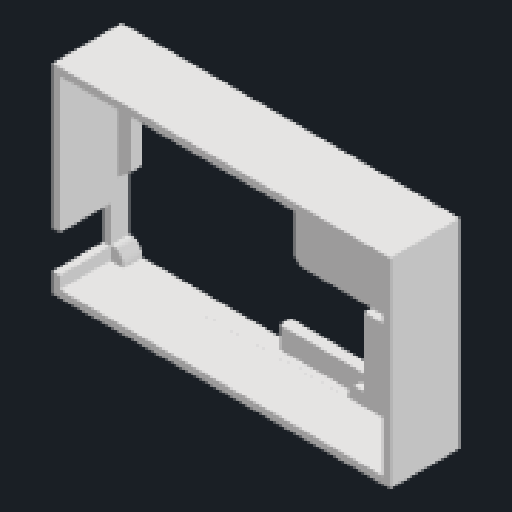
# Autodesk Inventor part: Buttom_case
Saved by Autodesk Inventor 2026.2 (Build 302298000, 298)
## iProperties
Created: 2026-04-11
Part Number: Buttom_case
Material: Generic
Document SubType Name: Modeling
Designer: Malthe Sennels
Density: 1 g/cm^3
Appearance: Default
Author: Malthe Sennels
Autodesk Inventor part; units mm, degrees
ref_plane "YZ Plane" through (0, 0, 0) normal (1, 0, 0) x (0, 1, 0)
ref_plane "XZ Plane" through (0, 0, 0) normal (0, 1, 0) x (-1, 0, 0)
sketch "Sketch1" plane through (0, 0, 0) normal (0, 0, 1) x (1, 0, 0)
  line L0 (139.954, -59.944) -> (184.404, -59.944)
  arc A0 (136.4, -63.498) -> (139.954, -59.944) centre (136.4, -59.944) ccw
  line L1 (136.398, -104.648) -> (136.4, -63.498)
  arc A1 (139.952, -108.202) -> (136.398, -104.648) centre (136.398, -108.202) ccw
  line L2 (198.6031, -108.1771) -> (139.952, -108.202)
  arc A2 (202.184, -104.6232) -> (198.6031, -108.1771) centre (202.1571, -108.1771) ccw
  line L3 (187.185, -59.444) -> (139.4128, -59.444)
  arc A3 (135.9, -62.9568) -> (139.4128, -59.444) centre (136.4, -59.944) ccw
  line L4 (135.9, -62.9568) -> (135.898, -105.1892)
  arc A4 (139.4108, -108.7022) -> (135.898, -105.1892) centre (136.398, -108.202) ccw
  line L5 (139.4108, -108.7022) -> (199.1442, -108.6768)
  arc A5 (202.1802, -105.1231) -> (199.1442, -108.6768) centre (202.1571, -108.1771) ccw
  line L6 (187.185, -59.444) -> (224.685, -59.444)
  line L7 (224.685, -59.444) -> (224.685, -105.1231)
  line L8 (224.685, -105.1231) -> (202.1802, -105.1231)
  line L9 (133.9, -57.444) -> (226.685, -57.444)
  line L10 (226.685, -57.444) -> (226.685, -110.6768)
  line L11 (226.685, -110.6768) -> (133.9, -110.6768)
  line L12 (133.9, -110.6768) -> (133.9, -57.444)
  line L13 (224.685, -105.1231) -> (206.185, -105.1231)
  line L14 (206.185, -105.1231) -> (206.185, -86.9231)
  line L15 (206.185, -86.9231) -> (224.685, -86.9231)
  line L16 (224.685, -86.9231) -> (224.685, -105.1231)
  line L17 (225.185, -101.396) -> (225.185, -85.896)
  line L18 (224.685, -59.444) -> (221.285, -59.444)
  line L19 (221.285, -59.444) -> (221.285, -67.444)
  line L20 (221.285, -67.444) -> (224.685, -67.444)
  line L21 (224.685, -67.444) -> (224.685, -59.444)
  point P0 (0, 0)
extrude "Extrusion1" add sketch "Sketch1" against normal blind 2 contours L6 L7 L20 L19 | L7 L8 L14 L15 | L9 L10 L11 L12
sketch "Sketch2" plane through (0, 0, -2) normal (0, 0, -1) x (-1, 0, 0)
  line L0 (-226.685, -110.6768) -> (-133.9, -110.6768) projected
  line L1 (-133.9, -110.6768) -> (-133.9, -57.444) projected
  line L2 (-133.9, -57.444) -> (-226.685, -57.444) projected
  line L3 (-226.685, -57.444) -> (-226.685, -110.6768) projected
  line L4 (-221.285, -59.444) -> (-139.4128, -59.444) projected
  arc A0 (-139.4128, -59.444) -> (-135.9, -62.9568) centre (-136.4, -59.944) ccw projected
  line L5 (-135.9, -62.9568) -> (-135.898, -105.1892) projected
  arc A1 (-135.898, -105.1892) -> (-139.4108, -108.7022) centre (-136.398, -108.202) ccw projected
  line L6 (-139.4108, -108.7022) -> (-199.1442, -108.6768) projected
  arc A2 (-199.1442, -108.6768) -> (-202.1802, -105.1231) centre (-202.1571, -108.1771) ccw projected
  line L7 (-202.1802, -105.1231) -> (-206.185, -105.1231) projected
  line L8 (-206.185, -105.1231) -> (-206.185, -86.9231) projected
  line L9 (-206.185, -86.9231) -> (-224.685, -86.9231) projected
  line L10 (-224.685, -86.9231) -> (-224.685, -67.444) projected
  line L11 (-206.185, -101.9751) -> (-181.6826, -101.9751)
  line L12 (-181.6826, -101.9751) -> (-181.6854, -108.6843)
  line L13 (-177.0715, -59.444) -> (-182.7923, -64.1474)
  line L14 (-182.7923, -64.1474) -> (-182.7923, -84.0815)
  line L15 (-182.7923, -84.0815) -> (-185.4081, -86.9231)
  line L16 (-185.4081, -86.9231) -> (-206.185, -86.9231)
  line L17 (-135.8997, -70.5788) -> (-139.4108, -73.1836)
  line L18 (-139.4108, -73.1836) -> (-139.4108, -87.5874)
  line L19 (-139.4108, -87.5874) -> (-135.8987, -90.4582)
  line L20 (-182.7923, -79.0709) -> (-188.2357, -79.0709)
  arc A3 (-190.4025, -77.0764) -> (-188.2357, -79.0709) centre (-188.2357, -76.8967) ccw
  line L21 (-190.4025, -77.0764) -> (-190.4025, -68.8146)
  arc A4 (-187.5463, -65.9584) -> (-190.4025, -68.8146) centre (-187.5463, -68.8146) ccw
  line L22 (-187.5463, -65.9584) -> (-182.7923, -65.9584)
  line L23 (-226.685, -57.444) -> (-221.285, -57.444)
  line L24 (-221.285, -57.444) -> (-221.285, -65.444)
  line L25 (-221.285, -65.444) -> (-226.685, -65.444)
  line L26 (-226.685, -65.444) -> (-226.685, -57.444)
  line L27 (-224.685, -67.444) -> (-221.285, -67.444) projected
  line L28 (-221.285, -67.444) -> (-221.285, -59.444) projected
  point P0 (0, 0)
  dimension "d47" = 5.4
  dimension "d48" = 8
  constraints: 32 end point, 7 point on line, 4 horizontal, 4 perpendicular, 4 point on circle, 3 tangent, 2 centre point, 2 parallel, 2 vertical
  measures "d47" distance of L24.end L25.end
  measures "d48" distance of L23.end L24.end
extrude "Extrusion2" add sketch "Sketch2" along normal blind 3 contours L3 L25 L28 L27 L10 L9 L8 L7 A2 L6 A1 L5 A0 L4 L24 L2 L1 L0 | L3 L2 L24 L25 | L24 L4 L13 L14 L22 A4 L21 A3 L20 L15 L16 L9 L10 L27 L28 | L5 L19 L18 L17 | L11 L12 L6 A2 L7 L8
sketch "Sketch3" plane through (0, 0, 0) normal (0, 0, 1) x (1, 0, 0)
  line L0 (133.9, -110.6768) -> (226.685, -110.6768) projected
  line L1 (226.685, -110.6768) -> (226.685, -57.444) projected
  line L2 (226.685, -57.444) -> (133.9, -57.444) projected
  line L3 (133.9, -57.444) -> (133.9, -110.6768) projected
  line L4 (139.4128, -59.444) -> (221.285, -59.444) projected
  line L5 (224.685, -67.444) -> (224.685, -86.9231) projected
  line L6 (224.685, -86.9231) -> (206.185, -86.9231) projected
  line L7 (206.185, -86.9231) -> (206.185, -105.1231) projected
  line L8 (206.185, -105.1231) -> (202.1802, -105.1231) projected
  arc A0 (202.1802, -105.1231) -> (199.1442, -108.6768) centre (202.1571, -108.1771) ccw projected
  line L9 (199.1442, -108.6768) -> (139.4108, -108.7022) projected
  arc A1 (139.4108, -108.7022) -> (135.898, -105.1892) centre (136.398, -108.202) ccw projected
  line L10 (135.898, -105.1892) -> (135.9, -62.9568) projected
  arc A2 (135.9, -62.9568) -> (139.4128, -59.444) centre (136.4, -59.944) ccw projected
  line L11 (133.9, -57.444) -> (226.685, -57.444)
  line L12 (226.685, -57.444) -> (226.685, -110.6768)
  line L13 (226.685, -110.6768) -> (133.9, -110.6768)
  line L14 (133.9, -110.6768) -> (133.9, -57.444)
  line L15 (135.9, -59.444) -> (224.685, -59.444)
  line L16 (224.685, -59.444) -> (224.685, -108.7022)
  line L17 (224.685, -108.7022) -> (135.9, -108.7022)
  line L18 (135.9, -108.7022) -> (135.9, -59.444)
  line L19 (135.989, -96.1155) -> (132.989, -96.1155) projected
  line L20 (135.989, -104.9155) -> (132.989, -104.9155) projected
  line L21 (135.989, -95.6155) -> (132.989, -95.6155)
  line L22 (135.989, -105.4155) -> (132.989, -105.4155)
  line L23 (133.3303, -95.6155) -> (137.6479, -95.6155)
  line L24 (137.6479, -95.6155) -> (137.6479, -105.4155)
  line L25 (137.6479, -105.4155) -> (133.3303, -105.4155)
  line L26 (133.3303, -105.4155) -> (133.3303, -95.6155)
  line L27 (226.685, -57.444) -> (221.285, -57.444)
  line L28 (221.285, -57.444) -> (221.285, -65.444)
  line L29 (221.285, -65.444) -> (226.685, -65.444)
  line L30 (226.685, -65.444) -> (226.685, -57.444)
  line L31 (221.285, -59.444) -> (221.285, -67.444) projected
  line L32 (221.285, -67.444) -> (224.685, -67.444) projected
  point P0 (0, 0)
  point P1 (135.9, -105.4155)
  point P2 (133.9, -105.4155)
  point P3 (133.9, -95.6155)
  point P4 (135.8984, -95.6155)
  point P5 (224.685, -59.444)
  point P6 (221.904, -86.9231)
  point P7 (135.9, -105.1889)
  point P8 (135.9, -95.6155)
  point P9 (221.285, -59.444)
  point P10 (135.898, -104.9155)
  point P11 (135.9, -104.9155)
  dimension "d12" = 0.5
  dimension "d13" = 0.5
  dimension "d45" = 5.4
  dimension "d46" = 8
  constraints: 36 end point, 10 parallel, 4 horizontal, 4 perpendicular, 2 point on line, 1 point on circle
  measures "d12" distance between parallel lines of L19 L21
  measures "d13" distance between parallel lines of L20 L22
  measures "d45" distance of L29.end L28.end
  measures "d46" distance of L28.end L27.end
extrude "Extrusion3" add sketch "Sketch3" along normal blind 15 from surface at 0 contours L3 L22 L18 L17 L16 L5 L29 L1 L0 | L29 L16 L15 L28 L2 L1 | L22 L25 A1 L17 L18 | L29 L28 L15 L16 | L16 L32 L31 L29 | L28 L4 L15 L18 L10 L21 L3 L2 | A2 L18 L15
sketch "Sketch4" plane through (0, 0, -5) normal (0, 0, -1) x (-1, 0, 0)
  line L0 (-133.9, -110.6768) -> (-133.9, -57.444) projected
  line L1 (-133.9, -57.444) -> (-226.685, -57.444) projected
  line L2 (-226.685, -57.444) -> (-226.685, -110.6768) projected
  line L3 (-226.685, -110.6768) -> (-133.9, -110.6768) projected
  arc A0 (-139.4128, -59.444) -> (-135.9, -62.9568) centre (-136.4, -59.944) ccw projected
  line L4 (-135.9, -62.9568) -> (-135.8997, -70.5788) projected
  line L5 (-135.8997, -70.5788) -> (-139.4108, -73.1836) projected
  line L6 (-139.4108, -73.1836) -> (-139.4108, -87.5874) projected
  line L7 (-139.4108, -87.5874) -> (-135.8987, -90.4582) projected
  line L8 (-135.8987, -90.4582) -> (-135.898, -105.1892) projected
  arc A1 (-135.898, -105.1892) -> (-139.4108, -108.7022) centre (-136.398, -108.202) ccw projected
  line L9 (-139.4108, -108.7022) -> (-181.6854, -108.6843) projected
  line L10 (-181.6854, -108.6843) -> (-181.6826, -101.9751) projected
  line L11 (-181.6826, -101.9751) -> (-206.185, -101.9751) projected
  line L12 (-206.185, -101.9751) -> (-206.185, -86.9231) projected
  line L13 (-206.185, -86.9231) -> (-185.4081, -86.9231) projected
  line L14 (-185.4081, -86.9231) -> (-182.7923, -84.0815) projected
  line L15 (-182.7923, -84.0815) -> (-182.7923, -79.0709) projected
  line L16 (-182.7923, -79.0709) -> (-188.2357, -79.0709) projected
  arc A2 (-190.4025, -77.0764) -> (-188.2357, -79.0709) centre (-188.2357, -76.8967) ccw projected
  line L17 (-190.4025, -77.0764) -> (-190.4025, -68.8146) projected
  arc A3 (-187.5463, -65.9584) -> (-190.4025, -68.8146) centre (-187.5463, -68.8146) ccw projected
  line L18 (-187.5463, -65.9584) -> (-182.7923, -65.9584) projected
  line L19 (-182.7923, -65.9584) -> (-182.7923, -64.1474) projected
  line L20 (-182.7923, -64.1474) -> (-177.0715, -59.444) projected
  line L21 (-177.0715, -59.444) -> (-139.4128, -59.444) projected
  point P0 (0, 0)
extrude "Extrusion4" add sketch "Sketch4" along normal blind 2 contours L3 L2 L1 L0 | A0 L4 L5 L6 L7 L8 A1 L9 L10 L11 L12 L13 L14 L15 L16 A2 L17 A3 L18 L19 L20 L21
sketch "Sketch5" plane through (133.9, -105.4155, 0) normal (-1, 0, 0) x (0, 0, 1)
  line L0 (8.585, 34.6765) -> (8.585, 37.2165) projected
  line L1 (8.585, 11.8165) -> (8.585, 14.3565) projected
  line L2 (6.585, 30.3855) -> (22, 30.3855)
  line L3 (22, 30.3855) -> (22, 18.3855)
  line L4 (22, 18.3855) -> (6.585, 18.3855)
  line L5 (6.585, 18.3855) -> (6.585, 30.3855)
  line L6 (6.585, 24.3855) -> (22, 24.3855)
  line L7 (6.585, 30.3855) -> (15, 30.3855)
  line L8 (15, 30.3855) -> (15, 18.3855)
  line L9 (15, 18.3855) -> (6.585, 18.3855)
  line L10 (15, 42.4587) -> (15, 9.8) projected
  line L11 (22, 18.3855) -> (22, 30.3855)
  line L12 (-8.585, -34.6765) -> (-8.585, -37.2165) projected
  line L13 (-8.585, -11.8165) -> (-8.585, -14.3565) projected
  line L14 (22, 18.3855) -> (24, 18.3855)
  line L15 (24, 18.3855) -> (24, 30.3855)
  line L16 (24, 30.3855) -> (22, 30.3855)
  line L17 (22, 30.3855) -> (22, 18.3855)
  point P0 (0, 105.4155)
  point P1 (14.2925, 18.3855)
  point P2 (16.8, 24.3855)
  point P3 (15, -30.5165)
  point P4 (15, 47.9715)
  point P5 (22, 30.3855)
  point P6 (15, 18.3855)
  dimension "d19" = 20.32
  dimension "d22" = 7
  dimension "d23" = 1.8
  dimension "d51" = 2
  dimension "d52" = 2
  constraints: 26 end point, 4 parallel, 4 perpendicular, 3 horizontal, 3 midpoint, 2 point on line
  measures "d19" distance of L0.start L1.end
  measures "d22" distance between parallel lines of L8 L3
  measures "d23" distance from line of point (16.8, 24.386) L8
  measures "d51" distance of L16.end L15.end
  measures "d52" distance between parallel lines of L0 L5
extrude "Extrusion5" cut sketch "Sketch5" against normal blind 16
fillet "Fillet1" radius 2 2 edges at (134.8994, -87.03, 6.585) (134.8997, -75.03, 6.585)
sketch "Sketch6" plane through (224.685, -86.9231, -2) normal (-1, 0, 0) x (0, 0, 1)
  circle A0 centre (20.335, -6.7229) radius 2.65 projected
  circle A1 centre (20.335, -6.7229) radius 3.35
  line L0 (17, -21.7791) -> (17, 19.4791) projected
  line L1 (17, 5.2771) -> (25, -2.7229)
  line L2 (25, -2.7229) -> (25, -10.7229)
  line L3 (25, -10.7229) -> (17, -18.7229)
  point P0 (2, 86.9231)
  point P1 (17, 27.4791)
  point P2 (17, -6.4062)
  point P3 (17, -7.0395)
  dimension "d27" = 0.7
  dimension "d28" = 45
  dimension "d29" = 45
  dimension "d30" = 8
  dimension "d31" = 4
  dimension "d32" = 4
  constraints: 6 end point, 2 point on line, 1 centre point, 1 parallel
  measures "d27" radial gap between concentric circles of A0 A1
  measures "d28" angle of L3 L0
  measures "d29" angle of L1 L0
  measures "d30" distance between parallel lines of L2 L0
  measures "d31" vertical distance of L2.end A0.centre
  measures "d32" vertical distance of L1.end A0.centre
extrude "Extrusion6" add sketch "Sketch6" against normal up to surface (2 mm away) contours A1 L0 L1 L2 L3
sketch "Sketch8" plane through (0, 0, 0) normal (0, 0, 1) x (1, 0, 0)
  line L0 (224.685, -108.7022) -> (224.685, -86.9231) projected
  line L1 (224.685, -108.7022) -> (220.685, -108.7022)
  line L2 (220.685, -108.7022) -> (220.685, -103.7022)
  line L3 (220.685, -103.7022) -> (224.685, -103.7022)
  line L4 (224.685, -103.7022) -> (224.685, -108.7022)
  point P0 (0, 0)
  dimension "d57" = 4
  dimension "d58" = 5
  constraints: 8 end point, 2 parallel, 1 horizontal, 1 perpendicular
  measures "d57" distance of L2.end L3.end
  measures "d58" distance of L1.end L2.end
extrude "Extrusion8" add sketch "Sketch8" along normal up to surface (15 mm away)
sketch "Sketch7" plane through (133.9, -57.444, 15) normal (0, 0, 1) x (1, 0, 0)
  circle A0 centre (1.3, -1.3) radius 1.8
  circle A1 centre (1.3, -1.3) radius 3.8
  line L0 (0, 0) -> (92.785, 0) projected
  line L1 (0, -53.2328) -> (0, 0) projected
  circle A2 centre (1.3, -51.9328) radius 1.8
  circle A3 centre (1.3, -51.9328) radius 3.8
  line L2 (92.785, -53.2328) -> (0, -53.2328) projected
  line L3 (0, -53.2328) -> (0, 0) projected
  line L4 (0, -47.9715) -> (3.7479, -47.9715) projected
  line L5 (92.785, -48.202) -> (90.785, -48.202) projected
  line L6 (0, -53.2328) -> (0, -47.9715) projected
  line L7 (92.785, -53.2328) -> (0, -53.2328) projected
  line L8 (92.785, -48.202) -> (92.785, -53.2328) projected
  line L9 (92.785, -35.8853) -> (90.785, -35.8853) projected
  line L10 (90.785, -24.202) -> (90.785, -10) projected
  line L11 (90.785, -24.202) -> (92.785, -24.202) projected
  line L12 (92.785, 0) -> (92.785, -24.202) projected
  line L13 (0, 0) -> (92.785, 0) projected
  line L14 (90.785, -36.5187) -> (92.785, -36.5187) projected
  line L15 (92.785, -35.8853) -> (92.785, -36.5187) projected
  line L16 (90.785, -36.5187) -> (90.785, -35.8853) projected
  line L17 (5.5107, -51.2582) -> (86.785, -51.2582) projected
  line L18 (1.9984, -38.1715) -> (0, -38.1715) projected
  line L19 (87.385, -2) -> (5.5128, -2) projected
  line L20 (87.385, -10) -> (87.385, -2) projected
  line L21 (90.785, -10) -> (87.385, -10) projected
  line L22 (0, -17.586) -> (0, 0) projected
  line L23 (2, -5.5128) -> (1.9994, -17.586) projected
  line L24 (0, -47.9715) -> (3.7479, -47.9715) projected
  line L25 (1.9988, -29.586) -> (0, -29.586) projected
  line L26 (0, -38.1715) -> (0, -29.586) projected
  line L27 (1.9988, -29.586) -> (1.9984, -38.1715) projected
  line L28 (0, -17.586) -> (1.9994, -17.586) projected
  arc A4 (2, -5.5128) -> (5.5128, -2) centre (2.5, -2.5) ccw projected
  arc A5 (5.5107, -51.2582) -> (3.7479, -47.9715) centre (2.498, -50.758) ccw projected
  circle A6 centre (91.485, -1.3) radius 1.8
  circle A7 centre (91.485, -1.3) radius 3.8
  line L29 (90.785, -46.2582) -> (90.785, -48.202) projected
  line L30 (86.785, -46.2582) -> (90.785, -46.2582) projected
  line L31 (86.785, -51.2582) -> (86.785, -46.2582) projected
  circle A8 centre (91.485, -51.9328) radius 1.8
  circle A9 centre (91.485, -51.9328) radius 3.8
  point P0 (-133.9, 57.444)
  point P1 (0, -17.455)
  point P2 (-20.1767, -7.6209)
  point P3 (0, -50.6878)
  point P4 (0, -53.1778)
  point P5 (0.055, -53.2328)
  point P6 (2.545, -53.2328)
  point P7 (0, -0.055)
  point P8 (0, -2.545)
  point P9 (2.545, 0)
  point P10 (0.055, 0)
  point P11 (2, -47.9715)
  point P12 (90.24, 0)
  point P13 (92.785, -2.545)
  point P14 (92.785, -50.7174)
  point P15 (92.785, -50.6878)
  point P16 (90.24, -53.2328)
  dimension "d35" = 3.6
  dimension "d36" = 2
  dimension "d37" = 1.3
  dimension "d38" = 1.3
  dimension "d39" = 3.6
  dimension "d40" = 2
  dimension "d41" = 1.3
  dimension "d42" = 1.3
  dimension "d53" = 3.6
  dimension "d54" = 2
  dimension "d55" = 1.3
  dimension "d56" = 1.3
  dimension "d61" = 3.6
  dimension "d62" = 2
  dimension "d63" = 1.3
  dimension "d64" = 1.3
  constraints: 8 centre point, 4 coincident, 1 midpoint
  measures "d35" diameter of A0
  measures "d36" radial gap between concentric circles of A1 A0
  measures "d37" distance from line of L0 A0.centre
  measures "d38" distance from line of L1 A0.centre
  measures "d39" diameter of A2
  measures "d40" radial gap between concentric circles of A3 A2
  measures "d41" distance from line of L2 A2.centre
  measures "d42" distance from line of L3 A2.centre
  measures "d53" diameter of A6
  measures "d54" radial gap between concentric circles of A6 A7
  measures "d55" distance from line of L12 A6.centre
  measures "d56" distance from line of L0 A6.centre
  measures "d61" diameter of A8
  measures "d62" radial gap between concentric circles of A8 A9
  measures "d63" horizontal distance of point (92.785, -50.717) A8.centre
  measures "d64" distance from line of L7 A8.centre
extrude "Extrusion7" cut sketch "Sketch7" against normal blind 25.6 contours A0 L1 L0 | A0 L1 L0 | L0 A6 L12 | L0 L12 A6 | L1 A2 L2 | L1 A2 L2 | A8 L8 L2 | A8 L8 L2
sketch "Sketch9" plane through (0, 0, -7) normal (0, 0, -1) x (-1, 0, 0)
  arc A0 (-136.445, -57.444) -> (-133.9, -59.989) centre (-135.2, -58.744) ccw projected
  arc A1 (-133.9, -108.1318) -> (-136.445, -110.6768) centre (-135.2, -109.3768) ccw projected
  arc A2 (-224.14, -110.6768) -> (-226.685, -108.1318) centre (-225.385, -109.3768) ccw projected
  arc A3 (-226.685, -59.989) -> (-224.14, -57.444) centre (-225.385, -58.744) ccw projected
  circle A4 centre (-225.385, -58.744) radius 3.8
  circle A5 centre (-225.385, -58.744) radius 1.8
  circle A6 centre (-225.385, -109.3768) radius 1.8
  circle A7 centre (-225.385, -109.3768) radius 3.8
  circle A8 centre (-135.2, -58.744) radius 1.8
  circle A9 centre (-135.2, -58.744) radius 3.8
  circle A10 centre (-135.2, -109.3768) radius 1.8
  circle A11 centre (-135.2, -109.3768) radius 3.8
  point P0 (0, 0)
  dimension "d65" = 2
  dimension "d66" = 2
  dimension "d67" = 2
  dimension "d68" = 2
  constraints: 8 coincident, 4 centre point, 12 other
  measures "d65" radial gap between concentric circles of A4 A3
extrude "Extrusion9" add sketch "Sketch9" against normal blind 5
sketch "Sketch10" plane through (0, 0, -7) normal (0, 0, -1) x (-1, 0, 0)
  arc A0 (-133.9, -62.3147) -> (-138.7707, -57.444) centre (-135.2, -58.744) ccw projected
  arc A1 (-138.7707, -110.6768) -> (-133.9, -105.8061) centre (-135.2, -109.3768) ccw projected
  arc A2 (-221.8143, -57.444) -> (-226.685, -62.3147) centre (-225.385, -58.744) ccw projected
  arc A3 (-226.685, -105.8061) -> (-221.8143, -110.6768) centre (-225.385, -109.3768) ccw projected
  circle A4 centre (-225.385, -58.744) radius 3.8
  circle A5 centre (-225.385, -109.3768) radius 3.8
  circle A6 centre (-135.2, -109.3768) radius 3.8
  circle A7 centre (-135.2, -58.744) radius 3.8
  point P0 (0, 0)
  point P1 (-226.685, -62.3147)
  point P2 (-133.9, -105.8061)
  constraints: 4 coincident, 12 other
extrude "Extrusion10" cut sketch "Sketch10" against normal blind 2
sketch "Sketch11" plane through (226.685, -97.646, 23) normal (1, 0, 0) x (0, 0, -1)
  line L0 (22.535, 12.6488) -> (22.535, 12.6488) projected
  line L1 (22.535, 13.5488) -> (22.535, 13.5488) projected
  line L2 (23.125, 13.5488) -> (23.125, 12.6488) projected
  point P0 (23, 97.646)
sketch "Sketch12" plane through (133.9, -95.6155, 15) normal (0, 0, 1) x (1, 0, 0)
  line L0 (1.9988, 8.5855) -> (0, 8.5855) projected
  line L1 (0, 0) -> (0, 8.5855) projected
  line L2 (1.9984, 0) -> (0, 0) projected
  line L3 (1.9988, 8.5855) -> (1.9984, 0) projected
  point P0 (-133.9, 95.6155)
ref_plane "Work Plane1" through (131.4, -113.1768, 18) normal (0, 0, 1) x (1, 0, 0)
extrude "Extrusion11" add sketch "Sketch12" along normal up to surface (3 mm away)
body "Solid1"
